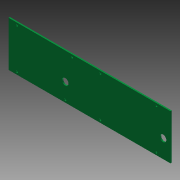
# Autodesk Inventor part: cRIO Electric Board 1764
Saved by Autodesk Inventor 2011 (Build 150239000, 239)
## iProperties
Category: FRC Parts
Manager: Ed Sparks
Company: FirstCadLibrary
Shininess: 64.0
Length Units: 11272
Angle Units: 11279
Time Units: 11290
Mass Units: 11286
Length Display Precision: 3
Angle Display Precision: 2
Compacted: True
Part Number: cRIO Electric Board 1764
Document SubType Name: Modeling
Created: 2008-12-13
Designer: Ed Sparks
Project: FIRST
Catalog Web Link: www.firstcadlibrary.com
Engineer: Ed Sparks
Material: Phenolic
Density: 5 g/cm^3
Density: 0.0
Volumn: 0.0
Area: 0.0
PropertySet Name: Model Information
Control State: 0
Master: False
Checked Out: False
Author: Ed Sparks
Keywords: FIRST
Autodesk Inventor part; units mm, degrees
ref_plane "YZ Plane" through (0, 0, 0) normal (1, 0, 0) x (0, 1, 0)
ref_plane "XZ Plane" through (0, 0, 0) normal (0, 1, 0) x (-1, 0, 0)
ref_plane "XY Plane" through (0, 0, 0) normal (0, 0, 1) x (1, 0, 0)
sketch "Sketch1" plane through (0, 0, 0) normal (0, 0, 1) x (1, 0, 0)
  line L0 (-136.525, 38.1) -> (136.525, 38.1)
  line L1 (136.525, 38.1) -> (136.525, -38.1)
  line L2 (136.525, -38.1) -> (-136.525, -38.1)
  line L3 (-136.525, -38.1) -> (-136.525, 38.1)
  line L4 (0, 0) -> (0, 38.1) construction
  line L5 (0, 0) -> (0, -38.1) construction
  line L6 (0, 0) -> (-136.525, 0) construction
  line L7 (0, 0) -> (136.525, 0) construction
  dimension "d0" = 273.05
  dimension "d1" = 76.2
  constraints: 16 end point, 4 midpoint, 2 collinear, 2 parallel, 1 horizontal, 1 perpendicular, 1 other
  measures "d0" distance of L0.start L0.end
  measures "d1" distance of L2.end L0.start
extrude "PCB" add sketch "Sketch1" along normal mid plane 2.2098
sketch "Sketch2" plane through (0, 0, 1.1049) normal (0, 0, 1) x (1, 0, 0)
  line L0 (-136.525, 38.1) -> (136.525, 38.1) projected
  line L1 (-136.525, -38.1) -> (-136.525, 38.1) projected
  line L2 (136.525, -38.1) -> (-136.525, -38.1) projected
  line L3 (-122.5042, 33.9217) -> (-122.5042, 38.1) construction
  line L4 (-122.5042, -33.9217) -> (-122.5042, -38.1) construction
  point P0 (-29.4894, 33.9217)
  point P1 (18.0848, 33.9217)
  point P2 (112.5728, 33.9217)
  point P3 (-40.9702, -33.9217)
  point P4 (18.0848, -33.9217)
  point P5 (112.5728, -33.9217)
  dimension "d4" = 67.8434
  dimension "d5" = 14.0208
  dimension "d6" = 93.0148
  dimension "d7" = 47.5742
  dimension "d8" = 94.488
  dimension "d9" = 81.534
  constraints: 6 horizontal alignment, 4 end point, 3 vertical alignment, 2 point on line, 2 vertical, 1 collinear
  measures "d4" distance of L4.start L3.start
  measures "d5" distance from line of L1 L3.start
  measures "d6" distance of point (-29.489, 33.922) L3.start
  measures "d7" distance of point (18.085, 33.922) point (-29.489, 33.922)
  measures "d8" distance of point (112.573, 33.922) point (18.085, 33.922)
  measures "d9" distance of point (-40.97, -33.922) L4.start
hole "Hole1" at (-122.5042, 33.9217, 1.1049) at (-122.5042, -33.9217, 1.1049) at (-29.4894, 33.9217, 1.1049) at (18.0848, 33.9217, 1.1049) at (112.5728, 33.9217, 1.1049) at (-40.9702, -33.9217, 1.1049) at (18.0848, -33.9217, 1.1049) at (112.5728, -33.9217, 1.1049) direction (0, 0, -1) diameter 3.429 end through all
sketch "Sketch3" plane through (0, 0, 1.1049) normal (0, 0, 1) x (1, 0, 0)
  circle A0 centre (18.0848, -33.9217) radius 1.7145 projected
  circle A1 centre (-40.9702, -33.9217) radius 1.7145 projected
  point P0 (-40.9702, -7.6581)
  point P1 (124.1298, -7.6581)
  dimension "d17" = 165.1
  dimension "d18" = 26.2636
  dimension "d19" = 59.055
  constraints: 1 horizontal alignment
  measures "d17" distance of point (124.13, -7.658) point (-40.97, -7.658)
  measures "d18" distance of point (-40.97, -7.658) A1.centre
  measures "d19" horizontal distance of point (-40.97, -7.658) A0.centre
hole "Hole2" at (-40.9702, -7.6581, 1.1049) at (124.1298, -7.6581, 1.1049) direction (0, 0, -1) diameter 11.0744 end through all
body "Solid1"
